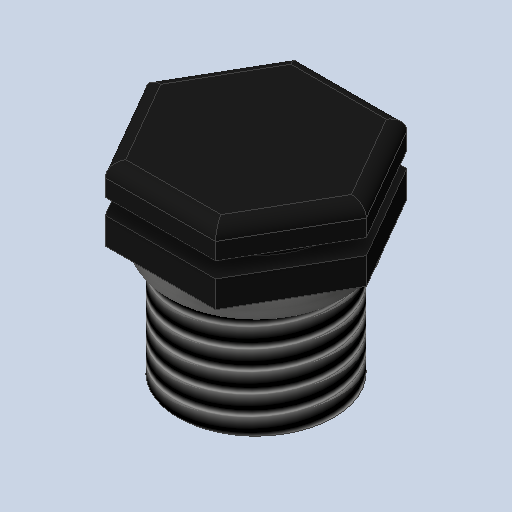
# Autodesk Inventor part: PMF100585
Saved by Autodesk Inventor 2024.2 (Build 282272000, 272)
## iProperties
Created: 2019-03-19
Part Number: PMF100585
Material: Generic
Document SubType Name: Modeling
Designer: lgnds
Density: 1 g/cm^3
Appearance: Default
Author: lgnds
Autodesk Inventor part; units mm, degrees
ref_plane "YZ Plane" through (0, 0, 0) normal (1, 0, 0) x (0, 1, 0)
ref_plane "XZ Plane" through (0, 0, 0) normal (0, 1, 0) x (-1, 0, 0)
sketch "Sketch1" plane through (0, 0, 0) normal (0, 0, 1) x (1, 0, 0)
  line L0 (0, 0) -> (6, 0)
  line L1 (6, 0) -> (6, 10)
  line L2 (6, 10) -> (8.5, 10)
  line L3 (8.5, 10) -> (8.5, 15.55)
  line L4 (8.5, 15.55) -> (0, 15.55)
  line L5 (0, 15.55) -> (0, 0)
  line L6 (0, -3.11) -> (0, 18.66) projected
  dimension "d0" = 10
  dimension "d1" = 5.55
  dimension "d2" = 8.5
  dimension "d3" = 6
  constraints: 12 end point, 5 perpendicular, 1 horizontal
  measures "d0" distance of L0.end L1.end
  measures "d1" distance of L2.end L3.end
  measures "d2" distance of L3.end L4.end
  measures "d3" distance between parallel lines of L5 L1
revolve "Revolution1" add sketch "Sketch1" angle 360 about axis through (0, -10, 0) along (0, 1, 0)
thread "Thread1" size "M12x1.5" class "6g" standard "ANSI Metric M Profile" full length
sketch "Sketch2" plane through (0, 0, 0) normal (0, 0, 1) x (1, 0, 0)
  line L0 (-8.5, 10) -> (8.5, 10) projected
  line L1 (-6, 10) -> (-6, 0) projected
  circle A0 centre (-6, 9) radius 1
  line L2 (0, -3.11) -> (0, 18.66) projected
  point P0 (0, 0)
  dimension "d8" = 2
  constraints: 1 centre point, 1 point on line, 1 tangent
  measures "d8" diameter of A0
revolve "Revolution2" add sketch "Sketch2" angle 360 about axis through (0, -10, 0) along (0, 1, 0) separate body
sketch "Sketch3" plane through (0, 15.55, 0) normal (0, 1, 0) x (1, 0, 0)
  circle A0 centre (0, 0) radius 8.5 projected
  line L0 (-8.5, 0) -> (-4.25, 7.3612)
  line L1 (-4.25, 7.3612) -> (4.25, 7.3612)
  line L2 (4.25, 7.3612) -> (8.5, 0)
  line L3 (8.5, 0) -> (4.25, -7.3612)
  line L4 (4.25, -7.3612) -> (-4.25, -7.3612)
  line L5 (-4.25, -7.3612) -> (-8.5, 0)
  constraints: 12 end point, 1 coincident, 1 horizontal, 1 horizontal alignment, 14 other
extrude "Extrusion1" cut sketch "Sketch3" against normal blind 10 contours L2 A0 | A0 L3 | L1 A0 | A0 L4 | L0 A0 | A0 L5 bodies 1
ref_plane "Work Plane1" through (-4.25, 12.05, 7.3612) normal (0, 1, 0) x (1, 0, 0)
sketch "Sketch4" plane through (-4.25, 12.05, 7.3612) normal (0, 1, 0) x (1, 0, 0)
  circle A0 centre (4.25, 7.3612) radius 6
  line L0 (0, 0) -> (8.5, 0) projected
  line L1 (-4.25, 7.3612) -> (0, 0) projected
  line L2 (0, 0) -> (8.5, 0) projected
  line L3 (8.5, 0) -> (12.75, 7.3612) projected
  line L4 (12.75, 7.3612) -> (8.5, 14.7224) projected
  line L5 (8.5, 14.7224) -> (0, 14.7224) projected
  line L6 (0, 14.7224) -> (-4.25, 7.3612) projected
  constraints: 1 centre point, 1 coincident
extrude "Extrusion2" cut sketch "Sketch4" along normal blind 1.2 bodies 1
fillet "Fillet2" radius 1 6 edges at (0, 15.55, -7.3612) (-6.375, 15.55, -3.6806) (-6.375, 15.55, 3.6806) (0, 15.55, 7.3612) (6.375, 15.55, 3.6806) (6.375, 15.55, -3.6806)
body "Solid1"
body "Solid2"
